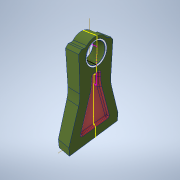
# Autodesk Inventor part: bearing holder
Saved by Autodesk Inventor 2021.1 (Build 251245000, 245)
## iProperties
Created: 2020-08-29
Part Number: bearing holder
Material: Aluminum 6061
Document SubType Name: Sheet Metal
Designer: Vamshi
Density: 2.7 g/cm^3
Sheet Metal Rule: Default
Appearance: Aluminum - Flat
Mass: 6551.43 g
Surface Area: 1895.37 cm^2
Volume: 2426.46 cm^3
Author: Vamshi
Autodesk Inventor part; units mm, degrees
ref_plane "YZ Plane" through (0, 0, 0) normal (1, 0, 0) x (0, 1, 0)
ref_plane "XZ Plane" through (0, 0, 0) normal (0, 1, 0) x (-1, 0, 0)
ref_plane "XY Plane" through (0, 0, 0) normal (0, 0, 1) x (1, 0, 0)
sketch "Sketch1" plane through (0, 0, 0) normal (0, 0, 1) x (1, 0, 0)
  line L0 (-116.84, -13.0015) -> (116.84, -13.0015)
  line L1 (116.84, -13.0015) -> (116.84, 25.0985)
  line L2 (-116.84, -13.0015) -> (-116.84, 25.0985)
  line L3 (0, -86.6615) -> (0, 428.9585) projected
  line L4 (-116.84, 25.0985) -> (-71.4229, 162.4275)
  line L5 (116.84, 25.0985) -> (71.4229, 162.4275)
  line L6 (-64.9999, 202.3045) -> (-64.9999, 324.8185)
  line L7 (64.9999, 202.3045) -> (64.9999, 324.8185)
  arc A0 (-65.1605, 181.3632) -> (-64.9999, 182.3601) centre (-68.1749, 182.3601) ccw
  arc A1 (-71.4229, 162.4275) -> (-64.9999, 202.3045) centre (-191.9999, 202.3045) ccw
  arc A2 (64.9999, 202.3045) -> (71.4229, 162.4275) centre (191.9999, 202.3045) ccw
  arc A3 (37.2472, 339.0425) -> (-37.2472, 339.0425) centre (0, 304.4985) ccw
  line L8 (-54.8399, 334.9785) -> (-46.559, 334.9785)
  line L9 (46.559, 334.9785) -> (54.8399, 334.9785)
  line L10 (0, 253.6985) -> (0, 227.7253)
  arc A4 (37.2472, 339.0425) -> (46.559, 334.9785) centre (46.559, 347.6785) ccw
  arc A5 (-46.559, 334.9785) -> (-37.2472, 339.0425) centre (-46.559, 347.6785) ccw
  arc A6 (37.2472, 339.0425) -> (46.559, 334.9785) centre (46.559, 347.6785) ccw
  line L11 (-54.8399, 334.9785) -> (-64.9999, 324.8185)
  line L12 (54.8399, 334.9785) -> (64.9999, 324.8185)
  point P0 (0, 0)
  point P1 (0, -13.0015)
  point P2 (-64.9999, 181.8487)
  point P3 (64.9999, 181.8487)
  point P4 (-64.9999, 334.9785)
  point P5 (64.9999, 334.9785)
  point P6 (-40.64, 334.9785)
  point P7 (40.64, 334.9785)
  dimension "d0" = 233.68
  dimension "d1" = 38.1
  dimension "d2" = 38.1
  dimension "d3" = 165.1
  dimension "d4" = 165.1
  dimension "d5" = 347.98
  dimension "d6" = 3.175
  dimension "d7" = 127
  dimension "d8" = 101.6
  dimension "d9" = 317.5
  dimension "d10" = 12.7
  dimension "d11" = 12.7
  dimension "d12" = 10.16
  dimension "d13" = 45
  dimension "d14" = 10.16
  dimension "d15" = 45
  constraints: 24 end point, 18 point on circle, 16 point on line, 12 tangent, 7 centre point, 3 horizontal, 3 vertical, 2 equal radius, 1 midpoint, 1 parallel, 1 perpendicular, 1 other
  measures "d0" distance of L0.start L0.end
  measures "d1" distance of L0.end L1.end
  measures "d2" distance of L0.start L2.end
  measures "d3" distance of L2.end point (-65, 181.849)
  measures "d4" distance of L1.end point (65, 181.849)
  measures "d5" distance from line of L0 point (-65, 334.979)
  measures "d6" radius of A0
  measures "d7" radius of A1
  measures "d8" diameter of A3
  measures "d9" distance from line of L0 A3.centre
  measures "d10" radius of A4
  measures "d11" radius of A5
  measures "d12" distance of L8.start point (-65, 334.979)
  measures "d13" angle of L8 L11
  measures "d14" distance of L9.end point (65, 334.979)
  measures "d15" angle of L9 L12
extrude "Extrusion1" add sketch "Sketch1" along normal mid plane 50.8
sketch "Sketch2" plane through (0, 0, 25.4) normal (0, 0, 1) x (1, 0, 0)
  arc A0 (37.2472, 339.0425) -> (-37.2472, 339.0425) centre (0, 304.4985) ccw projected
  circle A1 centre (0, 304.4985) radius 35.56
  line L0 (-62.9689, 44.3723) -> (-19.8142, 184.649)
  line L1 (62.9689, 44.3723) -> (19.8142, 184.649)
  line L2 (-58.1135, 37.7985) -> (58.1135, 37.7985)
  line L3 (116.84, 25.0985) -> (71.4229, 162.4275) projected
  line L4 (-71.4229, 162.4275) -> (-116.84, 25.0985) projected
  line L5 (-116.84, -13.0015) -> (116.84, -13.0015) projected
  line L6 (-9.1199, 240.9985) -> (9.1199, 240.9985)
  line L7 (-14.1999, 221.9921) -> (-14.1999, 235.9185)
  line L8 (14.1999, 221.9921) -> (14.1999, 235.9185)
  line L9 (-64.9999, 324.8185) -> (-64.9999, 202.3045) projected
  line L10 (64.9999, 202.3045) -> (64.9999, 324.8185) projected
  arc A2 (-19.8142, 184.649) -> (-14.1999, 221.9921) centre (-141.1999, 221.9921) ccw
  arc A3 (14.1999, 221.9921) -> (19.8142, 184.649) centre (141.1999, 221.9921) ccw
  arc A4 (-9.1199, 240.9985) -> (-14.1999, 235.9185) centre (-9.1199, 235.9185) ccw
  arc A5 (14.1999, 235.9185) -> (9.1199, 240.9985) centre (9.1199, 235.9185) ccw
  arc A6 (-62.9689, 44.3723) -> (-58.1135, 37.7985) centre (-58.1135, 42.8785) ccw
  arc A7 (58.1135, 37.7985) -> (62.9689, 44.3723) centre (58.1135, 42.8785) ccw
  point P0 (0, 0)
  point P1 (-64.9912, 37.7985)
  point P2 (-14.1999, 202.8985)
  point P3 (64.9912, 37.7985)
  point P4 (14.1999, 202.8985)
  dimension "d18" = 71.12
  dimension "d20" = 1.2
  dimension "d21" = 1.2
  dimension "d22" = 50.8
  dimension "d23" = 165.1
  dimension "d25" = 165.1
  dimension "d26" = 254
  dimension "d27" = 50.8
  dimension "d28" = 50.8
  dimension "d29" = 127
  dimension "d30" = 5.08
  constraints: 12 end point, 12 point on circle, 12 tangent, 8 point on line, 7 centre point, 4 equal radius, 2 horizontal, 2 perpendicular, 1 coincident
  measures "d18" diameter of A1
  measures "d20" angle of L4 L0
  measures "d21" angle of L3 L1
  measures "d22" distance between parallel lines of L5 L2
  measures "d23" vertical distance of point (-64.991, 37.799) point (-14.2, 202.899)
  measures "d25" vertical distance of point (64.991, 37.799) point (14.2, 202.899)
  measures "d26" distance between parallel lines of L5 L6
  measures "d27" distance between parallel lines of L9 L7
  measures "d28" distance between parallel lines of L10 L8
  measures "d29" radius of A2
  measures "d30" radius of A4
extrude "Extrusion2" cut sketch "Sketch2" against normal blind 50.8 contours A1
extrude "Extrusion3" cut sketch "Sketch2" against normal blind 10.16 contours L0 A2 L7 A4 L6 A5 L8 A3 L1 A7 L2 A6
fillet "Fillet1" radius 5.08 24 edges at (-62.1997, 39.8604, 15.24) (-41.3915, 114.5107, 15.24) (-15.6113, 203.1107, 15.24) (-14.1999, 228.9553, 15.24) (-12.712, 239.5106, 15.24) (0, 240.9985, 15.24) (12.712, 239.5106, 15.24) (14.1999, 228.9553, 15.24) (15.6113, 203.1107, 15.24) (41.3915, 114.5107, 15.24) (62.1997, 39.8604, 15.24) (0, 37.7985, 15.24) (-62.1997, 39.8604, 25.4) (-41.3915, 114.5107, 25.4) (-15.6113, 203.1107, 25.4) (-14.1999, 228.9553, 25.4) (-12.712, 239.5106, 25.4) (0, 240.9985, 25.4) (12.712, 239.5106, 25.4) (14.1999, 228.9553, 25.4) (15.6113, 203.1107, 25.4) (41.3915, 114.5107, 25.4) (62.1997, 39.8604, 25.4) (0, 37.7985, 25.4)
mirror "Mirror1" about plane through (0, 0, 0) normal (0, 0, 1) of "Extrusion3", "Fillet1"
fillet_without_effect "Fillet2"
sketch "Sketch3" plane through (-116.84, -13.0015, 25.4) normal (0, -1, 0) x (1, 0, 0)
  circle A0 centre (193.04, -25.4) radius 12.7
  circle A1 centre (40.64, -25.4) radius 12.7
  line L0 (116.84, -60.96) -> (116.84, 10.16) construction
  point P0 (116.84, -25.4)
  dimension "d37" = 25.4
  dimension "d38" = 25.4
  dimension "d39" = 152.4
  constraints: 2 centre point, 1 symmetric about line
  measures "d37" diameter of A0
  measures "d38" diameter of A1
  measures "d39" distance of A0.centre A1.centre
extrude "Extrusion4" cut sketch "Sketch3" against normal blind 50.8
thread "Thread1" size "M10x1.5" class "6H" standard "ANSI Metric M Profile" full length
thread "Thread2" size "M10x1.5" class "6H" standard "ANSI Metric M Profile" full length
sketch "Sketch4" plane through (0, 0, 0) normal (1, 0, 0) x (0, 1, 0)
  arc A0 (37.7985, 20.32) -> (32.7185, 25.4) centre (32.7185, 20.32) ccw projected
  arc A1 (37.7985, 20.32) -> (42.8785, 15.24) centre (42.8785, 20.32) ccw projected
  line L0 (42.8785, 15.24) -> (235.9185, 15.24) projected
  arc A2 (235.9185, 15.24) -> (240.9985, 20.32) centre (235.9185, 20.32) ccw projected
  arc A3 (246.0785, 25.4) -> (240.9985, 20.32) centre (246.0785, 20.32) ccw projected
  line L1 (246.0785, 25.4) -> (268.9385, 25.4) projected
  line L2 (268.9385, 25.4) -> (268.9385, -25.4) projected
  line L3 (268.9385, -25.4) -> (246.0785, -25.4) projected
  arc A4 (240.9985, -20.32) -> (246.0785, -25.4) centre (246.0785, -20.32) ccw projected
  arc A5 (240.9985, -20.32) -> (235.9185, -15.24) centre (235.9185, -20.32) ccw projected
  line L4 (235.9185, -15.24) -> (42.8785, -15.24) projected
  arc A6 (42.8785, -15.24) -> (37.7985, -20.32) centre (42.8785, -20.32) ccw projected
  arc A7 (32.7185, -25.4) -> (37.7985, -20.32) centre (32.7185, -20.32) ccw projected
  line L5 (32.7185, -25.4) -> (-13.0015, -25.4) projected
  line L6 (-13.0015, -25.4) -> (-13.0015, 25.4) projected
  line L7 (-13.0015, 25.4) -> (32.7185, 25.4) projected
  line L8 (340.0585, 25.4) -> (355.2985, 25.4) projected
  line L9 (355.2985, 25.4) -> (355.2985, -25.4) projected
  line L10 (355.2985, -25.4) -> (340.0585, -25.4) projected
  line L11 (340.0585, -25.4) -> (340.0585, 25.4) projected
  arc A8 (37.7985, 20.32) -> (32.7185, 25.4) centre (32.7185, 20.32) ccw projected
  arc A9 (37.7985, 20.32) -> (42.8785, 15.24) centre (42.8785, 20.32) ccw projected
  line L12 (42.8785, 15.24) -> (235.9185, 15.24) projected
  arc A10 (235.9185, 15.24) -> (240.9985, 20.32) centre (235.9185, 20.32) ccw projected
  arc A11 (246.0785, 25.4) -> (240.9985, 20.32) centre (246.0785, 20.32) ccw projected
  line L13 (246.0785, 25.4) -> (268.9385, 25.4) projected
  line L14 (268.9385, 25.4) -> (268.9385, -25.4) projected
  line L15 (268.9385, -25.4) -> (246.0785, -25.4) projected
  arc A12 (240.9985, -20.32) -> (246.0785, -25.4) centre (246.0785, -20.32) ccw projected
  arc A13 (240.9985, -20.32) -> (235.9185, -15.24) centre (235.9185, -20.32) ccw projected
  line L16 (235.9185, -15.24) -> (42.8785, -15.24) projected
  arc A14 (42.8785, -15.24) -> (37.7985, -20.32) centre (42.8785, -20.32) ccw projected
  arc A15 (32.7185, -25.4) -> (37.7985, -20.32) centre (32.7185, -20.32) ccw projected
  line L17 (32.7185, -25.4) -> (-13.0015, -25.4) projected
  line L18 (-13.0015, -25.4) -> (-13.0015, 25.4) projected
  line L19 (-13.0015, 25.4) -> (32.7185, 25.4) projected
  line L20 (340.0585, 25.4) -> (355.2985, 25.4) projected
  line L21 (355.2985, 25.4) -> (355.2985, -25.4) projected
  line L22 (355.2985, -25.4) -> (340.0585, -25.4) projected
  line L23 (340.0585, -25.4) -> (340.0585, 25.4) projected
  line L24 (324.8185, -25.4) -> (324.8185, 25.4) projected
  line L25 (202.3045, 25.4) -> (324.8185, 25.4) projected
  line L26 (202.3045, -25.4) -> (202.3045, 25.4) projected
  line L27 (324.8185, -25.4) -> (202.3045, -25.4) projected
  line L28 (324.8185, -25.4) -> (324.8185, 25.4) projected
  line L29 (202.3045, 25.4) -> (324.8185, 25.4) projected
  line L30 (202.3045, -25.4) -> (202.3045, 25.4) projected
  line L31 (324.8185, -25.4) -> (202.3045, -25.4) projected
  line L32 (268.9385, 25.4) -> (340.0585, 25.4) projected
  line L33 (340.0585, -25.4) -> (268.9385, -25.4) projected
  line L34 (268.9385, 25.4) -> (268.9385, -25.4)
  point P0 (0, 0)
  constraints: 2 end point, 1 vertical
sketch "Sketch7" plane through (0, 0, 0) normal (1, 0, 0) x (0, 1, 0)
  point P0 (0, 0)
chamfer "Chamfer1" distance 2.54 angle 45 1 edges at (-35.56, 304.4985, 25.4)
chamfer "Chamfer2" distance 2.54 angle 45 2 edges at (-38.1, 304.4985, 25.4) (-35.56, 304.4985, -25.4)
equation "\"d14\" = d12"
equation "\"d15\" = d13"
equation "\"BendRadius\" = Thickness"
equation "\"BendReliefWidth\" = Thickness"
equation "\"BendReliefDepth\" = 0.5 * Thickness"
equation "\"CornerReliefSize\" = 4 * Thickness"
equation "\"MinimumRemnant\" = 2 * Thickness"
equation "\"TransitionRadius\" = BendRadius"
equation "\"JacobiRadiusSize\" = BendRadius"
equation "\"GapSize\" = Thickness"
equation "\"Thickness\" = 3.048"
body "Solid1"
